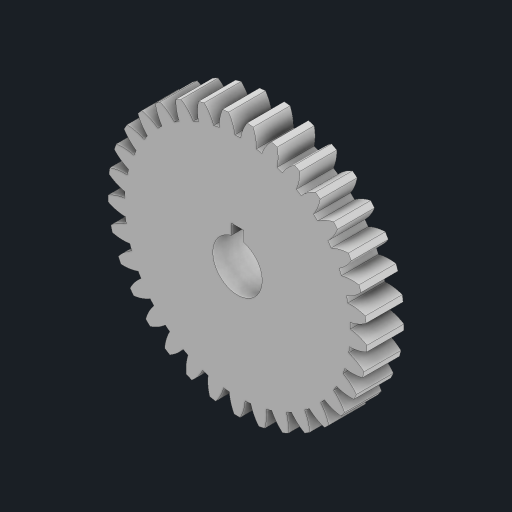
# Autodesk Inventor part: ENGRANAJE CONDUCTOR DE CAJA
Saved by Autodesk Inventor 2024.3 (Build 283343000, 343)
## iProperties
Created: 2024-06-16
Part Number: ENGRANAJE CONDUCTOR DE CAJA
Material: Generic
Document SubType Name: Modeling
Designer: Jhuliams
Density: 1 g/cm^3
Appearance: Default
Author: Jhuliams
Autodesk Inventor part; units mm, degrees
ref_plane "YZ Plane" through (0, 0, 0) normal (1, 0, 0) x (0, 1, 0)
ref_plane "XZ Plane" through (0, 0, 0) normal (0, 1, 0) x (-1, 0, 0)
ref_plane "XY Plane" through (0, 0, 0) normal (0, 0, 1) x (1, 0, 0)
sketch "Sketch1" plane through (0, 0, 0) normal (0, 0, 1) x (1, 0, 0)
  arc A0 (52.3587, -3.8498) -> (52.4806, -1.4281) centre (0, 0) ccw
  circle A1 centre (0, 0) radius 45.75
  line L0 (0, 0) -> (77.7116, 0) construction
  line L1 (0, 0) -> (65.7902, 0) construction
  arc A2 (52.4806, -1.4281) -> (45.7412, 0.8987) centre (43.7096, -15.909) ccw
  arc A3 (45.4197, -5.488) -> (52.3587, -3.8498) centre (45.0864, 11.4388) ccw
  arc A4 (52.141, 6.1288) -> (51.8025, 8.5297) centre (0, 0) ccw
  arc A5 (51.8025, 8.5297) -> (44.7445, 9.539) centre (45.9305, -7.3494) ccw
  arc A6 (45.6375, 3.2069) -> (52.141, 6.1288) centre (42.1068, 19.7647) ccw
  arc A7 (50.0389, 15.8858) -> (49.2521, 18.1792) centre (0, 0) ccw
  arc A8 (49.2521, 18.1792) -> (42.1306, 17.8346) centre (46.4914, 1.4758) ccw
  arc A9 (44.2058, 11.7859) -> (50.0389, 15.8858) centre (37.6054, 27.3763) ccw
  arc A10 (46.1282, 25.0686) -> (44.9216, 27.1717) centre (0, 0) ccw
  arc A11 (44.9216, 27.1717) -> (37.9941, 25.4856) centre (45.3719, 10.2477) ccw
  arc A12 (41.1765, 19.9389) -> (46.1282, 25.0686) centre (31.7448, 33.9984) ccw
  arc A13 (40.5504, 33.3454) -> (38.9675, 35.1821) centre (0, 0) ccw
  arc A14 (38.9675, 35.1821) -> (32.4843, 32.2154) centre (42.6126, 18.6492) ccw
  arc A15 (36.6589, 27.3713) -> (40.5504, 33.3454) centre (24.7369, 39.3918) ccw
  arc A16 (33.5069, 40.417) -> (31.6051, 41.921) centre (0, 0) ccw
  arc A17 (31.6051, 41.921) -> (25.8004, 37.7809) centre (38.3131, 26.3767) ccw
  arc A18 (30.8163, 33.8144) -> (33.5069, 40.417) centre (16.8349, 43.3614) ccw
  arc A19 (25.2524, 46.0279) -> (23.1003, 47.1447) centre (0, 0) ccw
  arc A20 (23.1003, 47.1447) -> (18.1841, 41.981) centre (32.629, 33.1508) ccw
  arc A21 (23.86, 39.0354) -> (25.2524, 46.0279) centre (8.3245, 45.7638) ccw
  arc A22 (16.0853, 49.9751) -> (13.7607, 50.6645) centre (0, 0) ccw
  arc A23 (13.7607, 50.6645) -> (9.9106, 44.6637) centre (25.7655, 38.7268) ccw
  arc A24 (16.0414, 42.8455) -> (16.0853, 49.9751) centre (-0.4868, 46.5122) ccw
  arc A25 (6.3367, 52.1162) -> (3.9237, 52.3532) centre (0, 0) ccw
  arc A26 (3.9237, 52.3532) -> (1.2788, 45.7321) centre (17.9708, 42.9031) ccw
  arc A27 (7.6429, 45.1071) -> (6.3367, 52.1162) centre (-9.2805, 45.5796) ccw
  arc A28 (-3.6408, 52.3736) -> (-6.0552, 52.1496) centre (0, 0) ccw
  arc A29 (-6.0552, 52.1496) -> (-7.3992, 45.1477) centre (9.5265, 45.5288) ccw
  arc A30 (-1.0318, 45.7384) -> (-3.6408, 52.3736) centre (-17.7388, 42.9995) ccw
  arc A31 (-13.4868, 50.7381) -> (-15.8151, 50.0613) centre (0, 0) ccw
  arc A32 (-15.8151, 50.0613) -> (-15.8097, 42.9315) centre (0.738, 46.5089) ccw
  arc A33 (-9.6692, 44.7165) -> (-13.4868, 50.7381) centre (-25.5559, 38.8654) ccw
  arc A34 (-22.8453, 47.2688) -> (-25.0035, 46.1636) centre (0, 0) ccw
  arc A35 (-25.0035, 46.1636) -> (-23.6489, 39.1637) centre (-8.0772, 45.8081) ccw
  arc A36 (-17.9571, 42.0786) -> (-22.8453, 47.2688) centre (-32.4494, 33.3266) ccw
  arc A37 (-31.3782, 42.0911) -> (-33.2881, 40.5974) centre (0, 0) ccw
  arc A38 (-33.2881, 40.5974) -> (-30.6333, 33.9804) centre (-16.6005, 43.4517) ccw
  arc A39 (-25.596, 37.9197) -> (-31.3782, 42.0911) centre (-38.1701, 26.5832) ccw
  arc A40 (-38.7769, 35.3921) -> (-40.3697, 33.5639) centre (0, 0) ccw
  arc A41 (-40.3697, 33.5639) -> (-36.5105, 27.5689) centre (-24.5238, 39.5248) ccw
  arc A42 (-32.3098, 32.3904) -> (-38.7769, 35.3921) centre (-42.5112, 18.8791) ccw
  arc A43 (-44.7742, 27.4139) -> (-45.9922, 25.3174) centre (0, 0) ccw
  arc A44 (-45.9922, 25.3174) -> (-41.0682, 20.161) centre (-31.5607, 34.1694) ccw
  arc A45 (-37.8559, 25.6904) -> (-44.7742, 27.4139) centre (-45.3159, 10.4926) ccw
  arc A46 (-49.1532, 18.445) -> (-49.9524, 16.1558) centre (0, 0) ccw
  arc A47 (-49.9524, 16.1558) -> (-44.1415, 12.0245) centre (-37.457, 27.579) ccw
  arc A48 (-42.0337, 18.0619) -> (-49.1532, 18.445) centre (-46.4827, 1.7269) ccw
  arc A49 (-51.7556, 8.8093) -> (-52.1072, 6.4103) centre (0, 0) ccw
  arc A50 (-52.1072, 6.4103) -> (-45.6195, 3.4534) centre (-41.9994, 19.9918) ccw
  arc A51 (-44.6923, 9.7805) -> (-51.7556, 8.8093) centre (-45.9695, -7.1012) ccw
  arc A52 (-52.4875, -1.1447) -> (-52.3787, -3.5669) centre (0, 0) ccw
  arc A53 (-52.3787, -3.5669) -> (-45.4486, -5.2426) centre (-45.0239, 11.6821) ccw
  arc A54 (-45.7357, 1.1457) -> (-52.4875, -1.1447) centre (-43.7949, -15.6727) ccw
  arc A55 (-51.3224, -11.0573) -> (-50.7571, -13.4152) centre (0, 0) ccw
  arc A56 (-50.7571, -13.4152) -> (-43.6351, -13.749) centre (-46.4211, 2.9501) ccw
  arc A57 (-45.126, -7.5305) -> (-51.3224, -11.0573) centre (-40.0374, -23.6777) ccw
  arc A58 (-48.3023, -20.5703) -> (-47.301, -22.7786) centre (0, 0) ccw
  arc A59 (-47.301, -22.7786) -> (-40.2446, -21.7586) centre (-46.1406, -5.8884) ccw
  arc A60 (-42.8853, -15.9346) -> (-48.3023, -20.5703) centre (-34.8328, -30.8269) ccw
  arc A61 (-43.5364, -29.3399) -> (-42.1353, -31.3187) centre (0, 0) ccw
  arc A62 (-42.1353, -31.3187) -> (-35.3995, -28.9817) centre (-44.1924, -14.5142) ccw
  arc A63 (-39.0947, -23.7627) -> (-43.5364, -29.3399) centre (-28.3693, -36.862) ccw
  arc A64 (-37.1971, -37.049) -> (-35.4468, -38.7269) centre (0, 0) ccw
  arc A65 (-35.4468, -38.7269) -> (-29.2749, -35.1574) centre (-40.6469, -22.6153) ccw
  arc A66 (-33.8911, -30.732) -> (-37.1971, -37.049) centre (-20.8805, -41.5648) ccw
  arc A67 (-29.5133, -43.4191) -> (-27.4771, -44.7354) centre (0, 0) ccw
  arc A68 (-27.4771, -44.7354) -> (-22.0923, -40.0624) centre (-35.6324, -29.8991) ccw
  arc A69 (-27.4625, -36.5906) -> (-29.5133, -43.4191) centre (-12.6369, -44.7653) ccw
  arc A70 (-20.7629, -48.2198) -> (-18.5143, -49.1271) centre (0, 0) ccw
  arc A71 (-18.5143, -49.1271) -> (-14.1112, -43.5194) centre (-29.33, -36.1023) ccw
  arc A72 (-20.0414, -41.1267) -> (-20.7629, -48.2198) centre (-3.9367, -46.3479) ccw
  arc A73 (-11.262, -51.2778) -> (-8.8824, -51.7431) centre (0, 0) ccw
  arc A74 (-8.8824, -51.7431) -> (-5.6201, -45.4035) centre (-21.9676, -41.0006) ccw
  arc A75 (-11.896, -44.1763) -> (-11.262, -51.2778) centre (4.9059, -46.2554) ccw
  arc A76 (-1.3541, -52.4825) -> (1.0706, -52.4891) centre (0, 0) ccw
  arc A77 (1.0706, -52.4891) -> (3.0741, -45.6466) centre (-13.8112, -44.4171) ccw
  arc A78 (-3.3206, -45.6293) -> (-1.3541, -52.4825) centre (13.5711, -44.491) ccw
  arc A79 (8.6028, -51.7904) -> (10.9849, -51.3379) centre (0, 0) ccw
  arc A80 (10.9849, -51.3379) -> (11.6572, -44.2399) centre (-5.1556, -46.2282) ccw
  arc A81 (5.3748, -45.4332) -> (8.6028, -51.7904) centre (21.7458, -41.1187) ccw
  arc A82 (18.2487, -49.2264) -> (20.5021, -48.3313) centre (0, 0) ccw
  arc A83 (20.5021, -48.3313) -> (19.819, -41.2343) centre (3.6863, -46.3685) ccw
  arc A84 (13.876, -43.595) -> (18.2487, -49.2264) centre (29.1346, -36.2602) ccw
  arc A85 (27.2351, -44.8832) -> (29.2784, -43.5778) centre (0, 0) ccw
  arc A86 (29.2784, -43.5778) -> (27.2645, -36.7384) centre (12.395, -44.8329) ccw
  arc A87 (21.8756, -40.1811) -> (27.2351, -44.8832) centre (35.4704, -30.0911) ccw
  arc A88 (35.2371, -38.9178) -> (36.9964, -37.2493) centre (0, 0) ccw
  arc A89 (36.9964, -37.2493) -> (33.7246, -30.9146) centre (20.6557, -41.677) ccw
  arc A90 (29.0846, -35.315) -> (35.2371, -38.9178) centre (40.5242, -22.8345) ccw
  arc A91 (41.9656, -31.5459) -> (43.3774, -29.5746) centre (0, 0) ccw
  arc A92 (43.3774, -29.5746) -> (38.9658, -23.9735) centre (28.1698, -37.0147) ccw
  arc A93 (35.2424, -29.1725) -> (41.9656, -31.5459) centre (44.1133, -14.7526) ccw
  arc A94 (47.1773, -23.0337) -> (48.1905, -20.8309) centre (0, 0) ccw
  arc A95 (48.1905, -20.8309) -> (42.7986, -16.166) centre (34.6658, -31.0146) ccw
  arc A96 (40.1265, -21.9756) -> (47.1773, -23.0337) centre (46.1081, -6.1375) ccw
  arc A97 (50.6839, -13.6891) -> (51.2619, -11.3344) centre (0, 0) ccw
  arc A98 (51.2619, -11.3344) -> (45.0846, -7.7741) centre (39.9089, -23.8936) ccw
  arc A99 (43.5603, -13.9845) -> (50.6839, -13.6891) centre (46.4364, 2.6994) ccw
  point P0 (-29.2749, -35.1574)
  point P1 (-27.4625, -36.5906)
  point P2 (-14.1112, -43.5194)
  point P3 (-11.896, -44.1763)
  point P4 (-5.6201, -45.4035)
  point P5 (-3.3206, -45.6293)
  point P6 (3.0741, -45.6466)
  point P7 (5.3748, -45.4332)
  point P8 (27.2645, -36.7384)
  point P9 (33.7246, -30.9146)
  point P10 (35.2424, -29.1725)
  point P11 (38.9658, -23.9735)
  point P12 (42.7986, -16.166)
  point P13 (43.5603, -13.9845)
  point P14 (45.0846, -7.7741)
  point P15 (45.4197, -5.488)
  point P16 (45.6375, 3.2069)
  point P17 (44.7445, 9.539)
  point P18 (42.1306, 17.8346)
  point P19 (37.9941, 25.4856)
  point P20 (36.6589, 27.3713)
  point P21 (25.8004, 37.7809)
  point P22 (23.86, 39.0354)
  point P23 (18.1841, 41.981)
  point P24 (16.0414, 42.8455)
  point P25 (7.6429, 45.1071)
  point P26 (1.2788, 45.7321)
  point P27 (-1.0318, 45.7384)
  point P28 (-7.3992, 45.1477)
  point P29 (-9.6692, 44.7165)
  point P30 (-15.8097, 42.9315)
  point P31 (-17.9571, 42.0786)
  point P32 (-23.6489, 39.1637)
  point P33 (-32.3098, 32.3904)
  point P34 (-36.5105, 27.5689)
  point P35 (-37.8559, 25.6904)
  point P36 (-41.0682, 20.161)
  point P37 (-42.0337, 18.0619)
  point P38 (-44.1415, 12.0245)
  point P39 (-44.6923, 9.7805)
  point P40 (-45.6195, 3.4534)
  point P41 (-45.7357, 1.1457)
  point P42 (-45.4486, -5.2426)
  point P43 (-45.126, -7.5305)
  point P44 (-43.6351, -13.749)
  point P45 (-42.8853, -15.9346)
  point P46 (-40.2446, -21.7586)
  point P47 (-35.3995, -28.9817)
  point P48 (-33.8911, -30.732)
  dimension "d2" = 91.5
  dimension "d1" = 105
  dimension "d7" = 360
  constraints: 198 point on circle, 99 centre point, 4 end point, 2 horizontal, 1 coincident, 334 other
  measures "d1" diameter of A0
extrude "Extrusion1" add sketch "Sketch1" along normal blind 15
sketch "Sketch2" plane through (0, 0, 15) normal (0, 0, 1) x (1, 0, 0)
  circle A0 centre (0, 0) radius 10
  line L0 (-2.5, 14) -> (2.5, 14)
  line L1 (2.5, 14) -> (2.5, -14)
  line L2 (2.5, -14) -> (-2.5, -14)
  line L3 (-2.5, -14) -> (-2.5, 14)
  line L4 (-2.5, 14) -> (2.5, -14) construction
  line L5 (2.5, 14) -> (-2.5, -14) construction
  line L6 (-2.5, 9.6825) -> (2.5, 9.6825) construction
  point P0 (-2.5, -9.6825)
  point P1 (2.5, -9.6825)
  dimension "d11" = 20
  dimension "d12" = 5
  dimension "d13" = 28
  constraints: 14 end point, 2 midpoint, 2 parallel, 2 point on circle, 2 point on line, 1 centre point, 1 coincident, 1 horizontal, 1 perpendicular
  measures "d11" diameter of A0
  measures "d12" distance of L1.end L2.end
  measures "d13" distance of L0.end L1.end
extrude "Extrusion2" cut sketch "Sketch2" against normal blind 15 contours A0 L1 | L1 A0 L3 | A0 L3 L0 L1 | L3 A0
body "Solid1"
